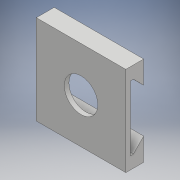
# Autodesk Inventor part: InnerFrame
Saved by Autodesk Inventor 2017 (Build 210142000, 142)
## iProperties
Created: 2016-05-22
Part Number: InnerFrame
Material: Generic
Document SubType Name: Modeling
Designer: Kurtis
Density: 1 g/cm^3
Appearance: Default
Author: Kurtis
Autodesk Inventor part; units mm, degrees
ref_plane "YZ Plane" through (0, 0, 0) normal (1, 0, 0) x (0, 1, 0)
ref_plane "XZ Plane" through (0, 0, 0) normal (0, 1, 0) x (-1, 0, 0)
ref_plane "XY Plane" through (0, 0, 0) normal (0, 0, 1) x (1, 0, 0)
sketch "Sketch1" plane through (0, 0, 0) normal (0, 0, 1) x (1, 0, 0)
  line L0 (-30, -6) -> (30, -6)
  line L1 (30, -6) -> (30, 6)
  line L2 (30, 6) -> (-30, 6)
  line L3 (-30, 6) -> (-30, -6)
  line L4 (-30, -6) -> (30, 6) construction
  line L5 (30, -6) -> (-30, 6) construction
  line L6 (30, 6) -> (25, 6) construction
  line L7 (-30, 6) -> (-25, 6) construction
  point P0 (0, 0)
  dimension "d0" = 60
  dimension "d1" = 12
  constraints: 16 end point, 2 midpoint, 2 parallel, 2 point on line, 1 horizontal, 1 perpendicular
  measures "d0" distance of L2.end L1.end
  measures "d1" distance of L1.end L0.end
extrude "Block" add sketch "Sketch1" along normal blind 60
sketch "Sketch2" plane through (30, -6, 0) normal (1, 0, 0) x (0, 0, -1)
  line L0 (0, 12) -> (-60, 12) projected
  line L1 (-30, 12) -> (-15.25, 12)
  line L2 (-30, 12) -> (-44.75, 12)
  line L3 (-30, 12) -> (-30, 3.1) construction
  line L4 (-30, 3.1) -> (-8.25, 3.1)
  line L5 (-30, 3.1) -> (-51.75, 3.1)
  line L6 (-51.75, 3.1) -> (-51.75, 5.1)
  line L7 (-8.25, 3.1) -> (-8.25, 5.1)
  line L8 (-8.25, 5.1) -> (-15.25, 12)
  line L9 (-51.75, 5.1) -> (-44.75, 12)
  point P0 (0, 6)
  dimension "d17" = 14.75
  dimension "d18" = 14.75
  dimension "d19" = 8.9
  dimension "d20" = 21.75
  dimension "d21" = 21.75
  dimension "d22" = 2
  dimension "d23" = 2
  constraints: 18 end point, 2 perpendicular, 2 point on line, 2 vertical, 1 horizontal, 1 midpoint
  measures "d17" distance of L1.start L1.end
  measures "d18" distance of L1.start L2.end
  measures "d19" distance of L1.start L3.end
  measures "d20" distance of L3.end L4.end
  measures "d21" distance of L3.end L5.end
  measures "d22" distance of L5.end L6.end
  measures "d23" distance of L4.end L7.end
extrude "Tripod Slot" cut sketch "Sketch2" against normal blind 60
hole "Hole1" at (0, -2.9, 30) direction (0, -1, 0) diameter 22.5 end through all
body "Solid1"
